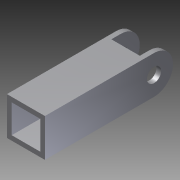
# Autodesk Inventor part: 8 ball pnumatic arm tube
Saved by Autodesk Inventor 2012 (Build 160160000, 160)
## iProperties
Created: 2013-10-08
Part Number: 8 ball pnumatic arm tube
Material: Default
Document SubType Name: Modeling
Designer: Bryce
Density: 1 g/cm^3
Author: Bryce
Autodesk Inventor part; units mm, degrees
ref_plane "YZ Plane" through (0, 0, 0) normal (1, 0, 0) x (0, 1, 0)
ref_plane "XZ Plane" through (0, 0, 0) normal (0, 1, 0) x (-1, 0, 0)
ref_plane "XY Plane" through (0, 0, 0) normal (0, 0, 1) x (1, 0, 0)
sketch "Sketch1" plane through (0, 0, 0) normal (0, 0, 1) x (1, 0, 0)
  line L0 (0, 0) -> (25.4, 0)
  line L1 (25.4, 0) -> (25.4, 25.4)
  line L2 (25.4, 25.4) -> (0, 25.4)
  line L3 (0, 25.4) -> (0, 0)
  line L4 (3.175, 3.175) -> (22.225, 3.175)
  line L5 (22.225, 3.175) -> (22.225, 22.225)
  line L6 (22.225, 22.225) -> (3.175, 22.225)
  line L7 (3.175, 22.225) -> (3.175, 3.175)
  dimension "d0" = 25.4
  dimension "d1" = 25.4
  dimension "d2" = 3.175
  dimension "d3" = 3.175
  dimension "d4" = 3.175
  dimension "d5" = 3.175
  constraints: 16 end point, 4 parallel, 2 horizontal, 2 perpendicular
  measures "d0" distance of L0.start L0.end
  measures "d1" distance of L2.end L0.start
  measures "d2" distance between parallel lines of L0 L4
  measures "d3" distance between parallel lines of L1 L5
  measures "d4" distance between parallel lines of L2 L6
  measures "d5" distance between parallel lines of L3 L7
extrude "Extrusion1" add sketch "Sketch1" along normal blind 85.725
sketch "Sketch2" plane through (25.4, 0, 0) normal (1, 0, 0) x (0, 0, -1)
  line L0 (-85.725, 25.4) -> (-85.725, 0) projected
  line L1 (0, 0) -> (-85.725, 0) projected
  line L2 (0, 0) -> (0, 25.4) projected
  line L3 (0, 25.4) -> (-85.725, 25.4) projected
  circle A0 centre (-12.7, 12.7) radius 4.7625
  arc A1 (-12.7, 0) -> (-12.7, 25.4) centre (-12.7, 12.7) ccw
  dimension "d8" = 9.525
  dimension "d9" = 12.7
  dimension "d10" = 12.7
  constraints: 3 tangent, 2 centre point, 2 point on circle, 2 point on line
  measures "d8" diameter of A0
  measures "d9" distance from line of L3 A0.centre
  measures "d10" distance from line of L2 A0.centre
extrude "Extrusion2" cut sketch "Sketch2" against normal blind 25.4 contours L3 L2 A1 | A1 L2 L1 | A0
sketch "Sketch3" plane through (0, 25.4, 85.725) normal (0, 1, 0) x (1, 0, 0)
  line L0 (0, 73.025) -> (25.4, 73.025) projected
  line L1 (3.175, 82.55) -> (22.225, 82.55)
  line L2 (22.225, 82.55) -> (22.225, 66.675)
  line L3 (22.225, 66.675) -> (3.175, 66.675)
  line L4 (3.175, 66.675) -> (3.175, 82.55)
  line L5 (0, 85.725) -> (0, 73.025) projected
  dimension "d13" = 19.05
  dimension "d14" = 3.175
  dimension "d17" = 15.875
  dimension "d18" = 6.35
  constraints: 8 end point, 2 parallel, 1 horizontal, 1 perpendicular
  measures "d13" distance of L1.start L1.end
  measures "d14" distance between parallel lines of L5 L4
  measures "d17" distance of L1.end L2.end
  measures "d18" distance between parallel lines of L3 L0
extrude "Extrusion3" cut sketch "Sketch3" against normal through all
equation "\"d2\" = d5"
equation "\"d3\" = d2"
equation "\"d5\" = d4"
equation "\"d10\" = d9"
body "Solid1"
